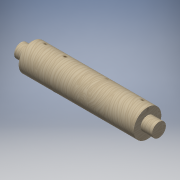
# Autodesk Inventor part: Roller
Saved by Autodesk Inventor 2019 (Build 230136000, 136)
## iProperties
Created: 2017-01-18
Part Number: Roller
Document SubType Name: Modeling
Designer: Administrator
Density: 1 g/cm^3
Mass: 5.93761 g
Surface Area: 22.9965 cm^2
Volume: 5.93761 cm^3
Material: Generic
Appearance: Wood (Grade B Plywood)
Author: Administrator
Autodesk Inventor part; units mm, degrees
ref_plane "YZ Plane" through (0, 0, 0) normal (1, 0, 0) x (0, 1, 0)
ref_plane "XZ Plane" through (0, 0, 0) normal (0, 1, 0) x (-1, 0, 0)
ref_plane "XY Plane" through (0, 0, 0) normal (0, 0, 1) x (1, 0, 0)
sketch "Sketch1" plane through (0, 0, 0) normal (0, 0, 1) x (1, 0, 0)
  line L0 (0, 0) -> (0, 6)
  line L1 (0, 6) -> (25, 6)
  line L2 (25, 6) -> (25, 3)
  line L3 (25, 3) -> (30, 3)
  line L4 (30, 3) -> (30, 0)
  line L5 (30, 0) -> (0, 0)
  dimension "d0" = 6
  dimension "d1" = 3
  dimension "d2" = 5
  dimension "d3" = 25
  constraints: 12 end point, 4 parallel, 1 perpendicular, 1 vertical, 1 other
  measures "d0" distance between parallel lines of L1 L5
  measures "d1" distance between parallel lines of L3 L5
  measures "d2" distance between parallel lines of L2 L4
  measures "d3" distance of L0.end L1.end
revolve "Revolution1" add sketch "Sketch1" angle 360 about axis through (30, 0, 0) along (-1, 0, 0)
mirror "Mirror1" about plane through (0, 3, 0) normal (-1, 0, 0) of "Revolution1"
body "Solid1"
